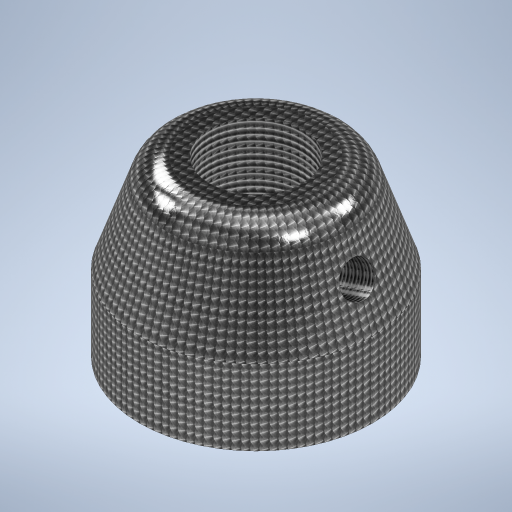
# Autodesk Inventor part: ClampingNut
Saved by Autodesk Inventor 2024 (Build 280153000, 153)
## iProperties
Created: 2023-11-09
Part Number: ClampingNut
Material: Polycarbonate, Clear
Document SubType Name: Modeling
Designer: Admin
Density: 1.2 g/cm^3
Appearance: Engine Turned
Author: Admin
Autodesk Inventor part; units mm, degrees
sketch "Sketch1" plane through (0, 0, 0) normal (0, 1, 0) x (-1, 0, 0)
  circle A0 centre (0, 0) radius 31
  dimension "d0" = 62
  constraints: 1 centre point, 1 coincident
  measures "d0" diameter of A0
extrude "Extrusion1" add sketch "Sketch1" along normal blind 20
sketch "Sketch2" plane through (0, 20, 0) normal (0, 1, 0) x (1, 0, 0)
  line L0 (0, 0) -> (31.1009, 0)
  circle A0 centre (0, 0) radius 31 projected
  constraints: 2 end point, 1 horizontal
ref_plane "Work Plane1" through (0, 46, 0) normal (0, 1, 0) x (-1, 0, 0)
ref_plane "Work Plane2" through (31, 0, 0) normal (1, 0, 0) x (0, 1, 0)
sketch "Sketch3" plane through (0, 46, 0) normal (0, 1, 0) x (-1, 0, 0)
  circle A0 centre (0, 0) radius 31 construction
  line L0 (0, 0) -> (-22, 0)
  circle A1 centre (0, 0) radius 22
  dimension "d5" = 22
  constraints: 2 end point, 1 coincident, 1 horizontal, 1 horizontal alignment, 2 other
  measures "d5" distance of L0.start L0.end
loft "Loft1" add profiles "Sketch3" section 1 edges at (31, 20, 0)
fillet "Fillet1" radius 8 1 edges at (22, 46, 0)
sketch "Sketch5" plane through (31, 0, 0) normal (1, 0, 0) x (0, 1, 0)
  line L0 (40.6169, -23.8634) -> (40.6169, 23.8634) projected
  line L1 (20, -31) -> (20, 31) projected
  point P0 (0, 0)
ref_plane "Work Plane3" through (31, 20, -31) normal (-0.9449861, -0.3271106, 0) x (0.3271106, -0.9449861, 0)
sketch "Sketch6" plane through (31, 20, -31) normal (-0.9449861, -0.3271106, 0) x (0.3271106, -0.9449861, 0)
  ellipse E0 centre (-29.6231, 31) end of major axis (-29.6231, 54.8634) minor radius 7.806 construction
  line L0 (34.5454, 31) -> (-68.4133, 31) construction
  point P0 (8.7593, 31)
  point P1 (-11.8171, 31)
  point P2 (-21.8171, 31)
  dimension "d11" = 10
  constraints: 2 point on line, 1 horizontal alignment, 1 other
  measures "d11" distance of point (-21.817, 31) point (-11.817, 31)
hole "Hole1" at (27.1345, 31.167, 0) direction (-0.9449861, -0.3271106, 0) diameter 9 depth 10 tip angle 118
thread "Thread1" size "M10x1" class "6H" standard "ANSI Metric M Profile" length 56
sketch "Sketch7" plane through (0, 46, 0) normal (0, 1, 0) x (1, 0, 0)
  circle A0 centre (0, 0) radius 12.5
  dimension "d21" = 25
  constraints: 1 centre point, 1 coincident
  measures "d21" diameter of A0
sketch "Sketch8" plane through (0, 0, 0) normal (0, -1, 0) x (1, 0, 0)
  circle A0 centre (0, 0) radius 12.5
  dimension "d22" = 25
  constraints: 1 centre point, 1 coincident
  measures "d22" diameter of A0
hole "Hole2" at (0, 0, 0) direction (0, 1, 0) diameter 25 end through all countersink diameter 28 countersink angle 45.49
thread "Thread2" size "M25x1.5" class "6H" standard "ANSI Metric M Profile" length 56
body "Solid1"
